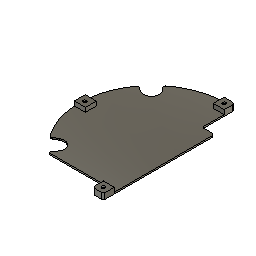
Compact_Robot_MB3 v1 (Autodesk Fusion 360 design; units mm, degrees)
Autodesk Fusion 360 part; units mm, degrees
note: some values were not read from the file. Set by a fixed rule: which sketch regions a step uses.
sketch "Esboço1" plane through (0, 0, 0) normal (0, 0, 1) x (1, 0, 0)
  line L0 (0, -37.25) -> (5.7315, -37.25)
  line L1 (0, -37.25) -> (-28.8244, -37.25)
  line L2 (13.7313, -37.25) -> (13.7313, -38.25)
  line L3 (13.7313, -38.25) -> (6.7313, -38.25)
  line L4 (6.7313, -38.25) -> (5.7315, -37.2502)
  line L5 (-33.6257, -26.0014) -> (-36.7371, -27.7066)
  line L6 (-27.7171, -34.088) -> (-28.9918, -35.3012)
  arc A0 (-31.1987, -35.48) -> (-30.9824, -35.4754) centre (-31.1987, -30.43) ccw
  arc A1 (-27.7171, -34.088) -> (-33.6257, -26.0014) centre (-31.1987, -30.43) ccw
  arc A2 (-31.1987, -35.2853) -> (-30.9824, -35.4754) centre (0, 0) ccw
  arc A3 (-28.8969, -37.1938) -> (-28.8244, -37.25) centre (0, 0) ccw
  arc A4 (-28.9918, -35.3012) -> (-28.8969, -37.1938) centre (-28.13, -36.2067) ccw
  arc A5 (-38.3557, -27.3358) -> (-36.7371, -27.7066) centre (-37.3378, -26.6104) ccw
  line L7 (13.7313, -45.25) -> (13.7313, -37.25)
  line L8 (13.7313, -30.43) -> (13.7313, 24.9988)
  line L9 (5.7315, -37.2502) -> (5.7315, -37.25)
  line L10 (13.7313, -37.25) -> (13.7313, -30.43)
  line L11 (6.7313, -38.25) -> (6.7313, -45.25)
  line L12 (6.7313, -45.25) -> (13.7313, -45.25)
  arc A6 (-34.0426, 26.2669) -> (-27.4054, 33.7737) centre (-31.1987, 30.44) ccw
  line L13 (-28.9198, 35.4969) -> (-27.4054, 33.7737)
  line L14 (-36.4461, 27.9049) -> (-34.0426, 26.2669)
  arc A7 (4.963, 46.8378) -> (-28.7437, 37.3123) centre (0, 0) ccw
  arc A8 (-38.1628, 27.6045) -> (-38.3557, -27.3358) centre (0, 0) ccw
  arc A9 (-28.7437, 37.3123) -> (-28.9198, 35.4969) centre (-27.9809, 36.3221) ccw
  arc A10 (-36.4461, 27.9049) -> (-38.1628, 27.6045) centre (-37.15, 26.8719) ccw
  line L15 (13.7313, 24.9988) -> (12.7371, 25.9986)
  line L16 (12.7371, 25.9986) -> (6.8571, 25.9986)
  line L17 (6.8571, 25.9986) -> (5.8601, 26.9956)
  line L18 (5.8601, 26.9956) -> (5.8601, 45.6356)
  line L19 (5.8601, 45.6356) -> (4.963, 46.8378)
  line L20 (5.8601, 40.1056) -> (-1.1399, 40.1056)
  line L21 (-1.1399, 40.1056) -> (-1.1399, 47.0862)
  line L22 (-46.9419, 3.8556) -> (-39.9419, 3.8556)
  line L23 (-39.9419, 3.8556) -> (-39.9419, -3.1444)
  line L24 (-39.9419, -3.1444) -> (-46.9949, -3.1444)
  circle A11 centre (-43.4419, 0) radius 2
  circle A12 centre (-43.4419, 0) radius 1.125
  circle A13 centre (10.2313, -41.75) radius 2
  circle A14 centre (10.2313, -41.75) radius 1.125
  circle A15 centre (2.3601, 43.6056) radius 2
  circle A16 centre (2.3601, 43.6056) radius 1.125
  dimension "d1" = 94.2
  dimension "d3" = 37.25
  dimension "d5" = 1
  dimension "d6" = 7
  dimension "d7" = 1.414
  dimension "d8" = 135
  dimension "d9" = 44.93
  dimension "d11" = 10.1
  dimension "d12" = 1.25
  dimension "d13" = 1.25
  dimension "d14" = 7
  dimension "d16" = 60.87
  dimension "d17" = 10.1
  dimension "d18" = 1.25
  dimension "d19" = 1.25
  dimension "d21" = 1.41
  dimension "d22" = 5.88
  dimension "d23" = 1.41
  dimension "d24" = 135
  dimension "d25" = 18.64
  dimension "d26" = 1.5
  dimension "d28" = 7
  dimension "d30" = 7
  dimension "d31" = 7
  dimension "d32" = 7.053
  dimension "d34" = 4
  dimension "d35" = 2.25
  dimension "d38" = 4
  dimension "d39" = 2.25
  dimension "d41" = 4
  dimension "d42" = 2.25
  constraint coincident A2.centre A3.centre
  constraint perpendicular L0 L7
  constraint perpendicular L0 L2
  constraint perpendicular L3 L7
  constraint coincident L8.start L7
  constraint concentric A2 A7
  constraint coincident L5.start A0
  constraint coincident L6.start A0
  constraint tangent L5 A0
  constraint tangent L6 A0
  constraint concentric A0 A1
  constraint concentric A2 A3
  constraint tangent A3 A4
  constraint tangent L6 A4
  constraint tangent L5 A5
  constraint tangent A5 A7
  constraint collinear L7 L8
  constraint perpendicular L0 L9
  constraint perpendicular L3 L11
  constraint perpendicular L11 L12
  constraint tangent A6 L13
  constraint tangent A6 L14
  constraint concentric A7 A8
  constraint tangent L13 A9
  constraint tangent A7 A9
  constraint tangent L14 A10
  constraint tangent A8 A10
  constraint perpendicular L8 L16
  constraint vertical L18
  constraint coincident L18 L20.start
  constraint perpendicular L18 L20
  constraint coincident A7 L21.end
  constraint perpendicular L20 L21
  constraint coincident A8 L22.start
  constraint perpendicular L22 L23
  constraint coincident A8 L24.end
  constraint perpendicular L23 L24
  constraint concentric A13 A14
  measures "d1" diameter of A7
  measures "d3" distance of A2.centre L0.start
  measures "d5" distance of L2.start L2.end
  measures "d6" distance of L2.end L3.end
  measures "d7" distance of L3.end L4.end
  measures "d8" angle of L0 L4
  measures "d9" distance of L8.start A0.centre
  measures "d11" diameter of A0
  measures "d12" radius of A4
  measures "d13" radius of A5
  measures "d14" distance of L3.end L11.end
  measures "d16" distance of A0.centre A6.centre
  measures "d17" diameter of A6
  measures "d18" radius of A9
  measures "d19" radius of A10
  measures "d21" distance of L8.end L15.end
  measures "d22" distance of L15.end L16.end
  measures "d23" distance of L16.end L17.end
  measures "d24" angle of L16 L17
  measures "d25" distance of L17.end L18.end
  measures "d26" distance of L18.end A7.start
  measures "d28" distance of L20.start L20.end
  measures "d30" distance of L22.start L22.end
  measures "d31" distance of L22.end L23.end
  measures "d32" distance of L23.end L24.end
  measures "d34" diameter of A11
  measures "d35" diameter of A12
  measures "d38" diameter of A13
  measures "d39" diameter of A14
  measures "d41" diameter of A15
  measures "d42" diameter of A16
extrude "Extrusão1" add sketch "Esboço1" along normal blind 1 contours L0 L1 L2 L3 L4 L5 L6 A1 A3 A4 A5 L7 L8 L10 A6 L13 L14 A7 A8 A9 A10 L15 L16 L17 L18 L20 L21 L22 L23 L24
extrude "Extrusão2" add sketch "Esboço1" along normal blind 3.75 contours A8 L22 L23 L24 | A11
extrude "Extrusão3" cut sketch "Esboço1" along normal blind 3 contours A11
extrude "Extrusão4" add sketch "Esboço1" along normal blind 3.75 contours L3 L7 L11 L12 | A13
extrude "Extrusão5" cut sketch "Esboço1" along normal blind 3 contours A13
extrude "Extrusão6" add sketch "Esboço1" along normal blind 3.75 contours A7 L18 L19 L20 L21 | A15
extrude "Extrusão7" cut sketch "Esboço1" along normal blind 3 contours A15
chamfer "Chanfro1" distance 1 angle 45 1 edges at (13.7313, -45.25, 1.875)
chamfer "Chanfro2" distance 1 angle 45 1 edges at (6.7313, -45.25, 1.875)
equation "d1 = ( 47.1 * 2 ) * 1 mm"
